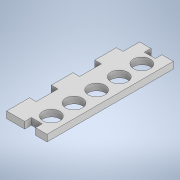
# Autodesk Inventor part: SupportV2
Saved by Autodesk Inventor 2020 (Build 240168000, 168)
## iProperties
Created: 2019-11-07
Part Number: SupportV2
Material: Générique
Document SubType Name: Modeling
Designer: erwan
Density: 1 g/cm^3
Appearance: Par défaut
Author: erwan
Autodesk Inventor part; units mm, degrees
ref_plane "YZ Plane" through (0, 0, 0) normal (1, 0, 0) x (0, 1, 0)
ref_plane "XZ Plane" through (0, 0, 0) normal (0, 1, 0) x (-1, 0, 0)
ref_plane "XY Plane" through (0, 0, 0) normal (0, 0, 1) x (1, 0, 0)
sketch "Esquisse1" plane through (0, 0, 0) normal (0, 1, 0) x (-1, 0, 0)
  line L0 (0, 0) -> (38, 0)
  line L1 (112, -419) -> (74, -419)
  line L2 (0, -419) -> (0, 0)
  line L3 (0, -419) -> (38, -419)
  circle A0 centre (45, -59.5) radius 28
  circle A1 centre (45, -134.5) radius 28
  circle A2 centre (45, -209.5) radius 28
  circle A3 centre (45, -284.5) radius 28
  circle A4 centre (45, -359.5) radius 28
  line L4 (112, 0) -> (74, 0)
  line L5 (0, 0) -> (38, 0)
  line L6 (0, -22) -> (0, 0)
  line L7 (38, 0) -> (38, -22)
  line L8 (38, -22) -> (74, -22)
  line L9 (74, -22) -> (74, 0)
  line L10 (74, 0) -> (112, 0)
  line L11 (38, -419) -> (38, -397)
  line L12 (38, -397) -> (74, -397)
  line L13 (74, -397) -> (74, -419)
  line L14 (38, -419) -> (0, -419)
  line L15 (112, 0) -> (134, 0)
  line L16 (134, 0) -> (134, -76)
  line L17 (134, -76) -> (112, -76)
  line L18 (112, -148) -> (134, -148)
  line L19 (134, -148) -> (134, -220)
  line L20 (134, -220) -> (112, -220)
  line L21 (112, -292) -> (134, -292)
  line L22 (134, -292) -> (134, -364)
  line L23 (134, -364) -> (112, -364)
  line L24 (112, -76) -> (112, -148)
  line L25 (112, -220) -> (112, -292)
  line L26 (112, -364) -> (112, -419)
  dimension "d0" = 112
  dimension "d1" = 419
  dimension "d8" = 56
  dimension "d9" = 56
  dimension "d10" = 56
  dimension "d11" = 56
  dimension "d12" = 56
  dimension "d19" = 38
  dimension "d21" = 22
  dimension "d23" = 38
  dimension "d26" = 76
  dimension "d28" = 72
  dimension "d29" = 72
  dimension "d30" = 72
  dimension "d31" = 72
  constraints: 54 end point, 9 parallel, 7 horizontal, 5 centre point, 3 perpendicular, 2 collinear, 1 vertical
  measures "d0" distance of L1.start L2.start
  measures "d1" distance of L4.start L1.start
  measures "d8" diameter of A0
  measures "d9" diameter of A1
  measures "d10" diameter of A2
  measures "d11" diameter of A3
  measures "d12" diameter of A4
  measures "d19" distance between parallel lines of L6 L7
  measures "d21" distance between parallel lines of L12 L1
  measures "d23" distance between parallel lines of L2 L11
  measures "d26" distance between parallel lines of L15 L17
  measures "d28" distance between parallel lines of L18 L20
  measures "d29" distance between parallel lines of L17 L18
  measures "d30" distance between parallel lines of L21 L23
  measures "d31" distance between parallel lines of L20 L21
extrude "Extrusion2" add sketch "Esquisse1" along normal blind 22
